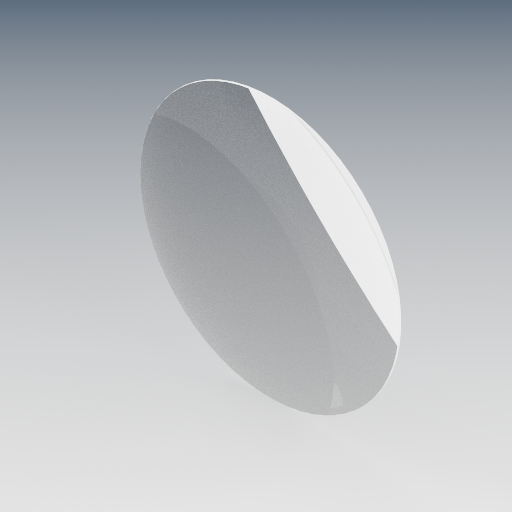
# Autodesk Inventor part: Plano convex Lens
Saved by Autodesk Inventor 2026 (Build 300175050, 175E)
## iProperties
Created: 2025-08-02
Part Number: Plano convex Lens
Material: Generic
Document SubType Name: Modeling
Designer: aman0
Density: 1 g/cm^3
Appearance: Default
Author: aman0
Autodesk Inventor part; units mm, degrees
ref_plane "YZ Plane" through (0, 0, 0) normal (1, 0, 0) x (0, 1, 0)
ref_plane "XZ Plane" through (0, 0, 0) normal (0, 1, 0) x (-1, 0, 0)
ref_plane "XY Plane" through (0, 0, 0) normal (0, 0, 1) x (1, 0, 0)
sketch "Sketch1" plane through (0, 0, 0) normal (0, 1, 0) x (-1, 0, 0)
  line L0 (0, 0) -> (-12.5, 0)
  circle A0 centre (0, -25) radius 27.9508
  line L1 (0, 0) -> (0, 2.9508)
  dimension "d0" = 12.5
  dimension "d1" = 25
  constraints: 4 end point, 2 point on circle, 1 centre point, 1 horizontal, 1 vertical
  measures "d0" distance of L0.start L0.end
  measures "d1" distance of L0.start A0.centre
revolve "Revolution1" add sketch "Sketch1" angle 360 about axis through (0, 0, 0) along (0, 0, 1) picked at (-7.0009, 0.542) contours L0 A0 L1
fillet "Fillet1" radius 0.1 1 edges at (-12.5, 0, 0)
body "Solid1"
